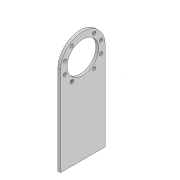
# Autodesk Inventor part: Axis 2 Arm
Saved by Autodesk Inventor 2020 (Build 240168000, 168)
## iProperties
Created: 2021-06-30
Part Number: Axis 2 Arm
Material: Generic
Document SubType Name: Modeling
Designer: Coy
Density: 1 g/cm^3
Appearance: Default
Author: Coy
Autodesk Inventor part; units mm, degrees
ref_plane "YZ Plane" through (0, 0, 0) normal (1, 0, 0) x (0, 1, 0)
ref_plane "XZ Plane" through (0, 0, 0) normal (0, 1, 0) x (-1, 0, 0)
ref_plane "XY Plane" through (0, 0, 0) normal (0, 0, 1) x (1, 0, 0)
sketch "Sketch1" plane through (0, 0, 0) normal (1, 0, 0) x (0, 1, 0)
  line L0 (150, 47.6174) -> (150, 47.7254)
  circle A0 centre (88.3156, 92.8725) radius 3
  circle A1 centre (31.6844, 92.8725) radius 3
  circle A2 centre (49.1844, 105.587) radius 3
  circle A3 centre (31.6844, 51.7275) radius 3
  circle A4 centre (70.8156, 39.013) radius 3
  circle A5 centre (88.3156, 51.7275) radius 3
  circle A6 centre (70.8156, 105.587) radius 3
  circle A7 centre (49.1844, 39.013) radius 3
  circle A8 centre (59.99, 72.3) radius 30 construction
  arc A9 (59.99, 32.3) -> (59.99, 112.3) centre (59.99, 72.3) ccw construction
  line L1 (-103.2, -308.2363) -> (-103.2, 417.5733)
  line L2 (-103.2, 112.3) -> (59.99, 112.3) construction
  line L3 (-103.2, 32.3) -> (59.99, 32.3) construction
  circle A10 centre (59.99, 72.3) radius 29
  line L4 (-103.2, 113.3) -> (59.99, 113.3)
  arc A11 (59.99, 31.3) -> (59.99, 113.3) centre (59.99, 72.3) ccw
  line L5 (59.99, 31.3) -> (-103.2, 31.3)
  point P0 (0, 0)
  point P1 (233, 72.3)
  point P2 (10, 134.109)
  point P3 (10, 10.5626)
  point P4 (-223, 72.3)
  point P5 (102.0387, 41.8672)
  point P6 (101.8384, 104.9787)
  point P7 (44.6465, 123.1195)
  point P8 (45.2345, 22.5467)
  dimension "d3" = 60
  dimension "d5" = 6
  dimension "d6" = 6
  dimension "d7" = 6
  dimension "d8" = 6
  dimension "d9" = 6
  dimension "d10" = 6
  dimension "d11" = 6
  dimension "d12" = 6
  dimension "d13" = 123.19
  dimension "d16" = 1
  dimension "d17" = 1
  constraints: 12 centre point, 12 end point, 4 point on circle, 2 perpendicular, 2 point on line, 2 tangent, 1 coincident, 1 vertical, 2 other
  measures "d3" diameter of A8
  measures "d5" diameter of A1
  measures "d6" diameter of A2
  measures "d7" diameter of A6
  measures "d8" diameter of A0
  measures "d9" diameter of A5
  measures "d10" diameter of A4
  measures "d11" diameter of A7
  measures "d12" diameter of A3
  measures "d13" distance edge to line of A9 L1
  measures "d16" radial gap between concentric circles of A8 A10
  measures "d17" radial gap between concentric circles of A9 A11
extrude "Extrusion1" add sketch "Sketch1" along normal blind 5
sketch "Sketch2" plane through (5, 0, 0) normal (1, 0, 0) x (0, 0, -1)
  point P0 (0, 0)
body "Solid1"
